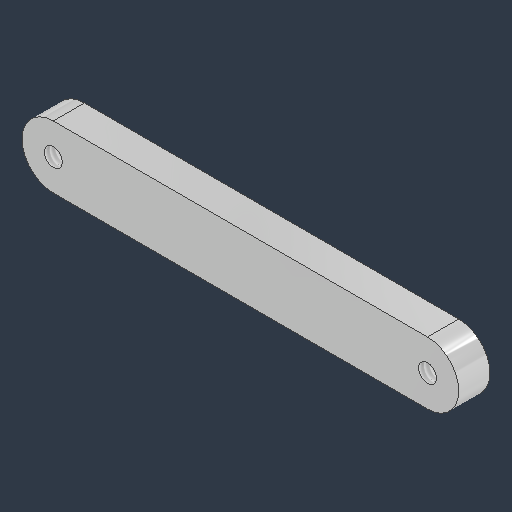
# Autodesk Inventor part: MOUNT,STRAP,BATTERY
Saved by Autodesk Inventor 2024.3 (Build 283343000, 343)
## iProperties
Created: 2025-01-26
Part Number: MOUNT,STRAP,BATTERY
Material: Aluminum 7075
Document SubType Name: Sheet Metal
Designer: Jthib
Density: 2.81 g/cm^3
Sheet Metal Rule: Default
Appearance: Aluminum - Polished
ILogicPurgeVersion: 0.0.0.0
ModelCat: Uncategorized
Author: Jthib
Autodesk Inventor part; units mm, degrees
ref_plane "YZ Plane" through (0, 0, 0) normal (1, 0, 0) x (0, 1, 0)
ref_plane "XZ Plane" through (0, 0, 0) normal (0, 1, 0) x (-1, 0, 0)
ref_plane "XY Plane" through (0, 0, 0) normal (0, 0, 1) x (1, 0, 0)
sketch "Sketch1" plane through (0, 0, 0) normal (0, 0, 1) x (1, 0, 0)
  line L0 (-44.45, -6.35) -> (44.45, -6.35)
  line L1 (44.45, -6.35) -> (44.45, 6.35)
  line L2 (44.45, 6.35) -> (-44.45, 6.35)
  line L3 (-44.45, 6.35) -> (-44.45, -6.35)
  line L4 (-44.45, -6.35) -> (44.45, 6.35) construction
  line L5 (44.45, -6.35) -> (-44.45, 6.35) construction
  point P0 (0, 0)
  dimension "d0" = 88.9
  dimension "d1" = 12.7
  measures "d0" distance of L1.end L2.end
  measures "d1" distance of L2.end L0.start
extrude "Plate1" add sketch "Sketch1" along normal mid plane 6.35
fillet "Corner Round1" radius 6.35 4 edges at (-44.45, -6.35, 0) (-44.45, 6.35, 0) (44.45, 6.35, 0) (44.45, -6.35, 0)
sketch "Sketch4" plane through (0, 0, 3.175) normal (0, 0, 1) x (1, 0, 0)
  arc A0 (-38.1, 6.35) -> (-38.1, -6.35) centre (-38.1, 0) ccw construction
  arc A1 (38.1, -6.35) -> (38.1, 6.35) centre (38.1, 0) ccw construction
  point P0 (0, 0)
  constraints: 2 coincident
hole "Hole1" at (-38.1, 0, 3.175) at (38.1, 0, 3.175) direction (0, 0, -1) diameter 3.683 end through all thread size "10-24 UNC" class "2B" standard "ANSI Unified Screw Threads"
equation "\"d29\" = Thickness"
equation "\"d2\" = Thickness"
equation "\"BendRadius\" = Thickness"
equation "\"BendReliefWidth\" = Thickness"
equation "\"BendReliefDepth\" = 0.5 * Thickness"
equation "\"CornerReliefSize\" = 4 * Thickness"
equation "\"MinimumRemnant\" = 2 * Thickness"
equation "\"TransitionRadius\" = BendRadius"
equation "\"JacobiRadiusSize\" = BendRadius"
equation "\"GapSize\" = Thickness"
equation "\"Thickness\" = 6.35"
body "Solid1"
